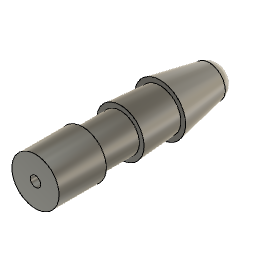
Screw-on-toy-insert v2 (Autodesk Fusion 360 design; units mm, degrees)
Autodesk Fusion 360 part; units mm, degrees
sketch "Sketch1" plane through (0, 0, 0) normal (1, 0, 0) x (0, 1, 0)
  line L0 (0, 0) -> (0, 12.5)
  line L1 (0, 12.5) -> (25, 12.5)
  line L2 (25, 12.5) -> (25, 10)
  line L3 (25, 10) -> (45, 10)
  line L4 (45, 10) -> (45, 12.5)
  line L5 (45, 12.5) -> (66, 12.5) construction
  line L6 (66, 12.5) -> (66, 11)
  line L7 (45, 12.5) -> (66, 11)
  line L8 (66, 12.5) -> (66, 13.5)
  line L9 (66, 13.5) -> (92, 13.5) construction
  line L10 (92, 13.5) -> (92, 8.5) construction
  line L11 (66, 13.5) -> (92, 8.5)
  line L12 (66, 13.5) -> (98, 13.5) construction
  line L13 (98, 13.5) -> (98, 0)
  arc A0 (98, 1.2362) -> (92, 8.5) centre (90.6031, 1.2362) ccw
  line L14 (98, 0) -> (0, 0)
  dimension "d1" = 12.5
  dimension "d2" = 25
  dimension "d4" = 20
  dimension "d6" = 21
  dimension "d9" = 26
  dimension "d10" = 5
  dimension "d11" = 13.5
  dimension "d12" = 12.5
  dimension "d13" = 10
  dimension "d14" = 11
  dimension "d15" = 32
  dimension "d16" = 7.3969
  constraint coincident L0.start L14.end
  constraint vertical L0
  constraint horizontal L1
  constraint perpendicular L1 L2
  constraint perpendicular L2 L3
  constraint perpendicular L3 L4
  constraint perpendicular L4 L5
  constraint perpendicular L5 L6
  constraint perpendicular L5 L8
  constraint perpendicular L8 L9
  constraint perpendicular L9 L10
  constraint perpendicular L8 L12
  constraint perpendicular L12 L13
  constraint tangent L13 A0
  constraint coincident L13 A0.start
  constraint tangent L11 A0
  constraint perpendicular L0 L14
  measures "d1" distance of L0.start L0.end
  measures "d2" distance of L0.end L1.end
  measures "d4" distance of L2.end L3.end
  measures "d6" distance of L4.end L5.end
  measures "d9" distance of L8.end L9.end
  measures "d10" distance of L9.end L10.end
  measures "d11" vertical distance of L0.start L8.end
  measures "d12" vertical distance of L0.start L4.end
  measures "d13" distance of L0.start L3
  measures "d14" vertical distance of L0.start L6.end
  measures "d15" distance of L8.end L12.end
  measures "d16" radius of A0
revolve "Revolve1" add sketch "Sketch1" angle 360 about axis through (0, 98, 0) along (0, -1, 0)
sketch "Sketch3" plane through (0, 0, 0) normal (0, -1, 0) x (1, 0, 0)
  circle A0 centre (0, 0) radius 12.5
  circle A1 centre (0, 0) radius 2.75
  dimension "d26" = 5.5
  constraint coincident A0.centre A1.centre
  measures "d26" diameter of A1
extrude "Extrude2" cut sketch "Sketch3" against normal blind 12.5 contours A1
equation "d1 = 25 mm / 2"
